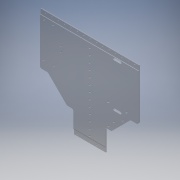
# Autodesk Inventor part: C15_TK_BatteryCrossStrut
Saved by Autodesk Inventor 2016 (Build 200138000, 138)
## iProperties
Created: 2016-01-20
Part Number: C15_TK_BatteryCrossStrut
Material: Polycarbonate, Clear
Document SubType Name: Modeling
Designer: TheeTimatahee
Density: 1.2 g/cm^3
Appearance: Polycarbonate - Clear
Mass: 810.244 g
Surface Area: 2322.62 cm^2
Volume: 675.204 cm^3
Author: TheeTimatahee
Autodesk Inventor part; units mm, degrees
ref_plane "YZ Plane" through (0, 0, 0) normal (1, 0, 0) x (0, 1, 0)
ref_plane "XZ Plane" through (0, 0, 0) normal (0, 1, 0) x (-1, 0, 0)
sketch "Sketch1" plane through (0, 0, 0) normal (0, 0, 1) x (1, 0, 0)
  line L0 (-196.85, -184.15) -> (196.85, -184.15)
  line L1 (196.85, -184.15) -> (196.85, 184.15)
  line L2 (196.85, 184.15) -> (-196.85, 184.15)
  line L3 (-196.85, 184.15) -> (-196.85, -184.15)
  line L4 (-196.85, -184.15) -> (196.85, 184.15) construction
  line L5 (196.85, -184.15) -> (-196.85, 184.15) construction
  point P0 (0, 0)
  dimension "d0" = 393.7
  dimension "d1" = 368.3
  constraints: 12 end point, 2 midpoint, 2 parallel, 1 horizontal, 1 perpendicular
  measures "d0" distance of L1.end L2.end
  measures "d1" distance of L0.end L1.end
extrude "Extrusion1" add sketch "Sketch1" along normal blind 6.35
sketch "Sketch2" plane through (0, 0, 6.35) normal (0, 0, 1) x (1, 0, 0)
  line L0 (-196.85, 184.15) -> (-196.85, -184.15) projected
  line L1 (-196.85, 165.1) -> (196.85, 165.1)
  line L2 (196.85, 165.1) -> (196.85, 184.15)
  line L3 (196.85, 184.15) -> (-196.85, 184.15)
  line L4 (-196.85, 184.15) -> (-196.85, 165.1)
  line L5 (-196.85, -184.15) -> (196.85, -184.15)
  line L6 (196.85, -184.15) -> (196.85, -165.1)
  line L7 (196.85, -165.1) -> (-196.85, -165.1)
  line L8 (-196.85, -165.1) -> (-196.85, -184.15)
  line L9 (196.85, -184.15) -> (196.85, 184.15) projected
  point P0 (0, 0)
  dimension "d4" = 330.2
  dimension "d5" = 19.05
  constraints: 16 end point, 4 parallel, 2 horizontal, 2 perpendicular, 1 collinear, 1 point on line
  measures "d4" distance between parallel lines of L7 L1
  measures "d5" distance between parallel lines of L3 L1
extrude "Extrusion2" cut sketch "Sketch2" against normal blind 2.54 contours L3 L2 L1 L0 | L7 L6 L5 L0
sketch "Sketch3" plane through (0, 0, 6.35) normal (0, 0, 1) x (1, 0, 0)
  line L0 (196.85, -184.15) -> (196.85, 165.1) projected
  line L1 (-196.85, 165.1) -> (-196.85, -165.1) projected
  line L2 (-63.5, -96.2801) -> (-63.5, -169.8131)
  line L3 (-196.85, -138.0631) -> (-196.85, -96.2801)
  line L4 (-169.0712, 11.938) -> (-156.3712, 11.938)
  line L5 (196.85, -184.15) -> (-196.85, -184.15) projected
  line L6 (-88.9, -96.2801) -> (-165.1, -20.0801)
  line L7 (-196.85, 184.15) -> (-196.85, -184.15) projected
  line L8 (-63.5, -96.2801) -> (-196.85, -96.2801)
  line L9 (-196.85, -96.2801) -> (-196.85, -7.3801)
  line L10 (-63.5, -169.8131) -> (-63.5, -184.15)
  line L11 (-63.5, -169.8131) -> (-63.5, -169.8131)
  line L12 (176.1744, -166.6059) -> (83.0336, -166.6059)
  line L13 (-176.1744, -166.6381) -> (-83.0336, -166.6381)
  line L14 (-176.1744, -102.6301) -> (-83.0336, -102.6301)
  line L15 (176.1744, -102.5979) -> (83.0336, -102.5979)
  line L16 (0, -214.5967) -> (0, 32.3311)
  line L17 (196.85, 165.1) -> (196.85, -165.1)
  line L18 (63.5, -96.2801) -> (63.5, -169.8131)
  line L19 (88.9, -96.2801) -> (165.1, -20.0801)
  line L20 (63.5, -96.2801) -> (196.85, -96.2801)
  line L21 (63.5, -169.8131) -> (63.5, -184.15)
  line L22 (63.5, -169.8131) -> (63.5, -169.8131)
  line L23 (196.85, -165.1) -> (196.85, -184.15)
  line L24 (196.85, -184.15) -> (196.85, 184.15) projected
  line L25 (196.85, -184.15) -> (63.5, -184.15)
  line L26 (-63.5, -184.15) -> (-196.85, -184.15)
  line L27 (-196.85, -184.15) -> (196.85, -184.15) projected
  line L28 (-196.85, -184.15) -> (-196.85, -138.0631)
  line L29 (-196.85, -20.0801) -> (196.85, -20.0801)
  line L30 (-196.85, -96.2801) -> (-196.85, -20.0801)
  line L31 (-196.85, -20.0801) -> (-165.1, -20.0801)
  line L32 (-165.1, -20.0801) -> (-165.1, -96.2801)
  line L33 (-165.1, -96.2801) -> (-196.85, -96.2801)
  line L34 (-196.85, -96.2801) -> (-196.85, -20.0801)
  point P0 (0, 0)
  point P1 (101.6, -190.5)
  dimension "d45" = 45
  dimension "d47" = 6.35
  dimension "d48" = 3.175
  dimension "d49" = 25.4
  dimension "d50" = 45
  dimension "d51" = 76.2
  constraints: 58 end point, 10 point on line, 9 horizontal, 7 symmetric about line, 5 collinear, 3 parallel, 3 perpendicular, 3 vertical, 13 other
  measures "d45" angle of L6 L8
  measures "d47" distance between parallel lines of L14 L8
  measures "d48" distance between parallel lines of L11 L13
  measures "d49" distance from line of L2 L6.start
  measures "d50" angle of L20 L19
  measures "d51" distance between parallel lines of L20 L29
extrude "Extrusion3" cut sketch "Sketch3" against normal through all contours L5 L21 L18 L20 L0 | L20 L19 L29 L0 | L5 L7 L1 L8 L2 L10 | L32 L8 L1 L29 | L6 L8 L32
fillet "Fillet1" radius 6.35 8 edges at (-88.9, -96.2801, 3.175) (-63.5, -96.2801, 3.175) (-165.1, -20.0801, 3.175) (-196.85, -20.0801, 3.175) (63.5, -96.2801, 3.175) (88.9, -96.2801, 3.175) (165.1, -20.0801, 3.175) (196.85, -20.0801, 3.175)
sketch "Sketch5" plane through (0, 0, 0) normal (0, 0, -1) x (-1, 0, 0)
  line L0 (63.5, -184.15) -> (63.5, -102.6301) projected
  line L1 (-196.85, 184.15) -> (196.85, 184.15) projected
  line L2 (196.85, 184.15) -> (196.85, -13.7301) projected
  point P0 (0, 0)
  point P1 (50.8, -177.8)
  point P2 (63.5, -163.4631)
  point P3 (177.8, 177.8)
  point P4 (152.4, 177.8)
  point P5 (127, 177.8)
  point P6 (101.6, 177.8)
  point P7 (76.2, 177.8)
  point P8 (50.8, 177.8)
  point P9 (25.4, 177.8)
  point P10 (0, 177.8)
  point P11 (-25.4, 177.8)
  point P12 (-50.8, 177.8)
  point P13 (-76.2, 177.8)
  point P14 (-101.6, 177.8)
  point P15 (-127, 177.8)
  point P16 (-152.4, 177.8)
  point P17 (-177.8, 177.8)
  point P18 (25.4, -177.8)
  point P19 (0, -177.8)
  point P20 (-25.4, -177.8)
  point P21 (-50.8, -177.8)
  dimension "d100" = 12.7
  dimension "d101" = 6.35
  dimension "d102" = 19.05
  dimension "d105" = 25.4
  dimension "d112" = 25.4
  constraints: 2 horizontal, 18 other
  measures "d100" distance from line of L0 point (50.8, -177.8)
  measures "d101" distance from line of L1 point (177.8, 177.8)
  measures "d102" distance from line of L2 point (177.8, 177.8)
  measures "d105" distance of point (177.8, 177.8) point (152.4, 177.8)
  measures "d112" distance of point (50.8, -177.8) point (25.4, -177.8)
hole "Hole2" at (-177.8, 177.8, 0) at (-152.4, 177.8, 0) at (-127, 177.8, 0) at (-101.6, 177.8, 0) at (-76.2, 177.8, 0) at (-50.8, 177.8, 0) at (-25.4, 177.8, 0) at (0, 177.8, 0) at (25.4, 177.8, 0) at (50.8, 177.8, 0) at (76.2, 177.8, 0) at (101.6, 177.8, 0) at (127, 177.8, 0) at (152.4, 177.8, 0) at (177.8, 177.8, 0) at (-50.8, -177.8, 0) at (-25.4, -177.8, 0) at (0, -177.8, 0) at (25.4, -177.8, 0) at (50.8, -177.8, 0) direction (0, 0, 1) diameter 4.1402 end through all
sketch "Sketch6" plane through (0, 0, 0) normal (0, 0, -1) x (-1, 0, 0)
  circle A0 centre (145.669, 153.0766) radius 2.4116 projected
  circle A1 centre (181.737, 153.0766) radius 2.4116 projected
  circle A2 centre (143.256, 13.1318) radius 2.4116 projected
  circle A3 centre (184.15, 13.1318) radius 2.4116 projected
  point P0 (0, 0)
hole "Hole3" at (-143.256, 13.1318, 0) at (-184.15, 13.1318, 0) at (-145.669, 153.0766, 0) at (-181.737, 153.0766, 0) direction (0, 0, 1) diameter 4.826 end through all
sketch "Sketch7" plane through (0, 0, 0) normal (0, 0, -1) x (-1, 0, 0)
  circle A0 centre (0, 184.15) radius 2.0701 projected
  line L0 (-9.6012, -190.5) -> (9.6012, -190.5) projected
  line L1 (9.6012, 190.5) -> (9.6012, -190.5) projected
  line L2 (9.6012, 190.5) -> (-9.6012, 190.5) projected
  line L3 (-9.6012, -190.5) -> (-9.6012, 190.5) projected
  circle A1 centre (0, 171.45) radius 2.0701 projected
  circle A2 centre (0, 146.05) radius 2.0701 projected
  circle A3 centre (0, 120.65) radius 2.0701 projected
  circle A4 centre (0, 95.25) radius 2.0701 projected
  circle A5 centre (0, 69.85) radius 2.0701 projected
  circle A6 centre (0, 44.45) radius 2.0701 projected
  circle A7 centre (0, 19.05) radius 2.0701 projected
  circle A8 centre (0, -6.35) radius 2.0701 projected
  circle A9 centre (0, -31.75) radius 2.0701 projected
  circle A10 centre (0, -57.15) radius 2.0701 projected
  circle A11 centre (0, -82.55) radius 2.0701 projected
  circle A12 centre (0, -107.95) radius 2.0701 projected
  circle A13 centre (0, -133.35) radius 2.0701 projected
  circle A14 centre (0, -158.75) radius 2.0701 projected
  circle A15 centre (0, -184.15) radius 2.0701 projected
  line L4 (-196.85, 165.1) -> (196.85, 165.1) projected
  line L5 (-36.3783, -2.794) -> (-171.9439, -2.794)
  line L6 (-123.19, -16.002) -> (-97.79, -16.002) construction
  line L7 (-123.19, -20.828) -> (-97.79, -20.828)
  line L8 (-97.79, -11.176) -> (-123.19, -11.176)
  arc A16 (-123.19, -11.176) -> (-123.19, -20.828) centre (-123.19, -16.002) ccw
  arc A17 (-97.79, -20.828) -> (-97.79, -11.176) centre (-97.79, -16.002) ccw
  line L9 (-123.19, 158.75) -> (-97.79, 158.75) construction
  line L10 (-123.19, 153.924) -> (-97.79, 153.924)
  line L11 (-97.79, 163.576) -> (-123.19, 163.576)
  arc A18 (-123.19, 163.576) -> (-123.19, 153.924) centre (-123.19, 158.75) ccw
  arc A19 (-97.79, 153.924) -> (-97.79, 163.576) centre (-97.79, 158.75) ccw
  line L12 (-110.49, 207.2769) -> (-110.49, -6.4547)
  line L13 (-196.85, -13.7301) -> (-196.85, 165.1) projected
  point P0 (0, 0)
  point P1 (-74.295, -2.794)
  point P2 (-146.685, -2.794)
  point P3 (-110.49, -16.002)
  point P4 (-110.49, 158.75)
  dimension "d118" = 72.39
  dimension "d119" = 13.208
  dimension "d120" = 4.826
  dimension "d121" = 25.4
  dimension "d122" = 23.495
  dimension "d123" = 4.826
  dimension "d124" = 25.4
  dimension "d127" = 6.35
  dimension "d128" = 86.36
  dimension "d129" = 165.1
  constraints: 20 end point, 8 point on circle, 8 tangent, 4 centre point, 4 point on line, 3 horizontal, 2 midpoint, 2 parallel, 1 vertical
  measures "d118" distance of point (-146.685, -2.794) point (-74.295, -2.794)
  measures "d119" distance from line of L5 point (-110.49, -16.002)
  measures "d120" radius of A17
  measures "d121" distance of L6.end L6.start
  measures "d122" horizontal distance of point (-74.295, -2.794) L6.end
  measures "d123" radius of A19
  measures "d124" distance of L9.start L9.end
  measures "d127" distance from line of L4 point (-110.49, 158.75)
  measures "d128" distance between parallel lines of L13 L12
  measures "d129" distance between parallel lines of L8 L10
extrude "Extrusion4" cut sketch "Sketch7" against normal through all contours L11 A19 L10 L12 | L12 L10 A18 L11 | A16 L8 A17 L7
hole "Hole4" at (74.295, -2.794, 0) at (146.685, -2.794, 0) direction (0, 0, 1) diameter 6.858 end through all
hole "Hole6" at (0, 146.05, 0) at (0, 120.65, 0) at (0, 95.25, 0) at (0, 69.85, 0) at (0, 44.45, 0) at (0, 19.05, 0) at (0, -6.35, 0) at (0, -31.75, 0) at (0, -57.15, 0) at (0, -82.55, 0) at (0, -107.95, 0) at (0, -133.35, 0) at (0, -158.75, 0) direction (0, 0, 1) diameter 5.1054 end through all clearance for "Flat Head Machine Screw (82)" size "#10" standard "Ansi Unified Screw Threads"
ref_plane "Work Plane1" through (0, 0, 3.175) normal (0, 0, -1) x (-1, 0, 0)
sketch "Sketch8" plane through (0, 0, 3.175) normal (0, 0, -1) x (-1, 0, 0)
  circle A0 centre (0, -133.35) radius 2.5527 projected
  circle A1 centre (0, -82.55) radius 2.5527 projected
  circle A2 centre (0, -31.75) radius 2.5527 projected
  circle A3 centre (0, 19.05) radius 2.5527 projected
  circle A4 centre (0, 69.85) radius 2.5527 projected
  circle A5 centre (0, 120.65) radius 2.5527 projected
  circle A6 centre (0, 146.05) radius 2.5527 projected
  circle A7 centre (0, 95.25) radius 2.5527 projected
  circle A8 centre (0, 44.45) radius 2.5527 projected
  circle A9 centre (0, -6.35) radius 2.5527 projected
  circle A10 centre (0, -57.15) radius 2.5527 projected
  circle A11 centre (0, -107.95) radius 2.5527 projected
  circle A12 centre (0, -158.75) radius 2.5527 projected
  circle A13 centre (145.669, 153.0766) radius 2.413 projected
  circle A14 centre (143.256, 13.1318) radius 2.413 projected
  circle A15 centre (184.15, 13.1318) radius 2.413 projected
  circle A16 centre (181.737, 153.0766) radius 2.413 projected
  circle A17 centre (-25.4, -177.8) radius 2.0701 projected
  circle A18 centre (25.4, -177.8) radius 2.0701 projected
  circle A19 centre (-177.8, 177.8) radius 2.0701 projected
  circle A20 centre (-127, 177.8) radius 2.0701 projected
  circle A21 centre (-76.2, 177.8) radius 2.0701 projected
  circle A22 centre (-25.4, 177.8) radius 2.0701 projected
  circle A23 centre (25.4, 177.8) radius 2.0701 projected
  circle A24 centre (76.2, 177.8) radius 2.0701 projected
  circle A25 centre (127, 177.8) radius 2.0701 projected
  circle A26 centre (177.8, 177.8) radius 2.0701 projected
  circle A27 centre (152.4, 177.8) radius 2.0701 projected
  circle A28 centre (101.6, 177.8) radius 2.0701 projected
  circle A29 centre (50.8, 177.8) radius 2.0701 projected
  circle A30 centre (0, 177.8) radius 2.0701 projected
  circle A31 centre (-50.8, 177.8) radius 2.0701 projected
  circle A32 centre (-101.6, 177.8) radius 2.0701 projected
  circle A33 centre (-152.4, 177.8) radius 2.0701 projected
  circle A34 centre (50.8, -177.8) radius 2.0701 projected
  circle A35 centre (0, -177.8) radius 2.0701 projected
  circle A36 centre (-50.8, -177.8) radius 2.0701 projected
  arc A37 (-196.85, -13.7301) -> (-190.5, -20.0801) centre (-190.5, -13.7301) ccw projected
  line L0 (-190.5, -20.0801) -> (-167.7303, -20.0801) projected
  arc A38 (-163.2401, -21.9399) -> (-167.7303, -20.0801) centre (-167.7303, -26.4301) ccw projected
  line L1 (-163.2401, -21.9399) -> (-90.7599, -94.4202) projected
  arc A39 (-90.7599, -94.4202) -> (-86.2697, -96.2801) centre (-86.2697, -89.9301) ccw projected
  line L2 (-86.2697, -96.2801) -> (-69.85, -96.2801) projected
  arc A40 (-63.5, -102.6301) -> (-69.85, -96.2801) centre (-69.85, -102.6301) ccw projected
  line L3 (-63.5, -102.6301) -> (-63.5, -184.15) projected
  line L4 (63.5, -184.15) -> (-63.5, -184.15) projected
  line L5 (63.5, -184.15) -> (63.5, -102.6301) projected
  arc A41 (69.85, -96.2801) -> (63.5, -102.6301) centre (69.85, -102.6301) ccw projected
  line L6 (69.85, -96.2801) -> (86.2697, -96.2801) projected
  arc A42 (86.2697, -96.2801) -> (90.7599, -94.4202) centre (86.2697, -89.9301) ccw projected
  line L7 (90.7599, -94.4202) -> (163.2401, -21.9399) projected
  arc A43 (167.7303, -20.0801) -> (163.2401, -21.9399) centre (167.7303, -26.4301) ccw projected
  line L8 (167.7303, -20.0801) -> (190.5, -20.0801) projected
  arc A44 (190.5, -20.0801) -> (196.85, -13.7301) centre (190.5, -13.7301) ccw projected
  line L9 (196.85, 184.15) -> (196.85, -13.7301) projected
  line L10 (-196.85, 184.15) -> (196.85, 184.15) projected
  line L11 (-196.85, -13.7301) -> (-196.85, 184.15) projected
  circle A45 centre (0, -133.35) radius 2.5527 projected
  circle A46 centre (0, -82.55) radius 2.5527 projected
  circle A47 centre (0, -31.75) radius 2.5527 projected
  circle A48 centre (0, 19.05) radius 2.5527 projected
  circle A49 centre (0, 69.85) radius 2.5527 projected
  circle A50 centre (0, 120.65) radius 2.5527 projected
  circle A51 centre (0, 146.05) radius 2.5527 projected
  circle A52 centre (0, 95.25) radius 2.5527 projected
  circle A53 centre (0, 44.45) radius 2.5527 projected
  circle A54 centre (0, -6.35) radius 2.5527 projected
  circle A55 centre (0, -57.15) radius 2.5527 projected
  circle A56 centre (0, -107.95) radius 2.5527 projected
  circle A57 centre (0, -158.75) radius 2.5527 projected
  circle A58 centre (145.669, 153.0766) radius 2.413 projected
  circle A59 centre (143.256, 13.1318) radius 2.413 projected
  circle A60 centre (184.15, 13.1318) radius 2.413 projected
  circle A61 centre (181.737, 153.0766) radius 2.413 projected
  arc A62 (-196.85, -13.7301) -> (-190.5, -20.0801) centre (-190.5, -13.7301) ccw projected
  line L12 (-196.85, -13.7301) -> (-196.85, 165.1) projected
  line L13 (-196.85, 165.1) -> (196.85, 165.1) projected
  line L14 (196.85, 165.1) -> (196.85, -13.7301) projected
  arc A63 (190.5, -20.0801) -> (196.85, -13.7301) centre (190.5, -13.7301) ccw projected
  line L15 (190.5, -20.0801) -> (167.7303, -20.0801) projected
  arc A64 (167.7303, -20.0801) -> (163.2401, -21.9399) centre (167.7303, -26.4301) ccw projected
  line L16 (163.2401, -21.9399) -> (90.7599, -94.4202) projected
  arc A65 (86.2697, -96.2801) -> (90.7599, -94.4202) centre (86.2697, -89.9301) ccw projected
  line L17 (86.2697, -96.2801) -> (69.85, -96.2801) projected
  arc A66 (69.85, -96.2801) -> (63.5, -102.6301) centre (69.85, -102.6301) ccw projected
  line L18 (63.5, -102.6301) -> (63.5, -165.1) projected
  line L19 (63.5, -165.1) -> (-63.5, -165.1) projected
  line L20 (-63.5, -165.1) -> (-63.5, -102.6301) projected
  arc A67 (-63.5, -102.6301) -> (-69.85, -96.2801) centre (-69.85, -102.6301) ccw projected
  line L21 (-69.85, -96.2801) -> (-86.2697, -96.2801) projected
  arc A68 (-90.7599, -94.4202) -> (-86.2697, -96.2801) centre (-86.2697, -89.9301) ccw projected
  line L22 (-90.7599, -94.4202) -> (-163.2401, -21.9399) projected
  arc A69 (-163.2401, -21.9399) -> (-167.7303, -20.0801) centre (-167.7303, -26.4301) ccw projected
  line L23 (-167.7303, -20.0801) -> (-190.5, -20.0801) projected
  line L24 (89.15, 101.9) -> (89.15, 107.9) projected
  line L25 (89.15, 101.9) -> (85.65, 101.9) projected
  line L26 (85.65, 60.9) -> (85.65, 101.9) projected
  line L27 (120.65, 60.9) -> (85.65, 60.9) projected
  line L28 (120.65, 110.9) -> (120.65, 60.9) projected
  line L29 (85.65, 110.9) -> (120.65, 110.9) projected
  line L30 (85.65, 107.9) -> (85.65, 110.9) projected
  line L31 (89.15, 107.9) -> (85.65, 107.9) projected
  circle A70 centre (113.65, 95.9) radius 2.15 projected
  circle A71 centre (113.65, 75.9) radius 2.15 projected
  point P0 (0, 0)
sketch "Sketch9" plane through (0, 0, 6.35) normal (0, 0, 1) x (1, 0, 0)
  arc A0 (168.4147, -77.5476) -> (161.6583, -77.5476) centre (165.0365, -77.5476) ccw projected
  line L0 (168.4147, -77.5476) -> (168.4147, -80.7226) projected
  arc A1 (161.6583, -80.7226) -> (168.4147, -80.7226) centre (165.0365, -80.7226) ccw projected
  line L1 (161.6583, -80.7226) -> (161.6583, -77.5476) projected
  line L2 (182.8165, -99.4551) -> (55.8165, -99.4551) projected
  line L3 (182.8165, -29.6051) -> (182.8165, -99.4551) projected
  line L4 (128.7395, -29.6051) -> (182.8165, -29.6051) projected
  line L5 (55.8165, -80.6663) -> (128.7395, -29.6051) projected
  line L6 (55.8165, -99.4551) -> (55.8165, -80.6663) projected
  circle A2 centre (97.0915, -61.3551) radius 2.5527 projected
  circle A3 centre (74.8665, -86.7551) radius 2.5527 projected
  circle A4 centre (132.0292, -39.1301) radius 2.5527 projected
hole "Hole7" at (132.0292, -39.1301, 6.35) at (97.0915, -61.3551, 6.35) at (74.8665, -86.7551, 6.35) direction (0, 0, -1) diameter 5.1054 end through all clearance for "Flat Head Machine Screw (82)" size "#10" standard "Ansi Unified Screw Threads"
hole "Hole8" at (-113.65, 75.9, 3.175) at (-113.65, 95.9, 3.175) direction (0, 0, 1) diameter 4.2926 end through all
sketch "Sketch10" plane through (0, 0, 6.35) normal (0, 0, 1) x (1, 0, 0)
  circle A0 centre (-113.65, 75.9) radius 2.1463 projected
  circle A1 centre (-113.65, 95.9) radius 2.1463 projected
  circle A2 centre (97.0915, -61.3551) radius 2.5527 projected
  circle A3 centre (132.0292, -39.1301) radius 2.5527 projected
  circle A4 centre (74.8665, -86.7551) radius 2.5527 projected
  circle A5 centre (0, -133.35) radius 2.5527 projected
  circle A6 centre (0, -82.55) radius 2.5527 projected
  circle A7 centre (0, -31.75) radius 2.5527 projected
  circle A8 centre (0, 19.05) radius 2.5527 projected
  circle A9 centre (0, 69.85) radius 2.5527 projected
  circle A10 centre (0, 120.65) radius 2.5527 projected
  circle A11 centre (0, 146.05) radius 2.5527 projected
  circle A12 centre (0, 95.25) radius 2.5527 projected
  circle A13 centre (0, 44.45) radius 2.5527 projected
  circle A14 centre (0, -6.35) radius 2.5527 projected
  circle A15 centre (0, -57.15) radius 2.5527 projected
  circle A16 centre (0, -107.95) radius 2.5527 projected
  circle A17 centre (0, -158.75) radius 2.5527 projected
  circle A18 centre (74.295, -2.794) radius 3.429 projected
  circle A19 centre (146.685, -2.794) radius 3.429 projected
  arc A20 (97.79, -11.176) -> (97.79, -20.828) centre (97.79, -16.002) ccw projected
  line L0 (97.79, -11.176) -> (123.19, -11.176) projected
  arc A21 (123.19, -20.828) -> (123.19, -11.176) centre (123.19, -16.002) ccw projected
  line L1 (123.19, -20.828) -> (97.79, -20.828) projected
  arc A22 (97.79, 163.576) -> (97.79, 153.924) centre (97.79, 158.75) ccw projected
  line L2 (97.79, 163.576) -> (123.19, 163.576) projected
  arc A23 (123.19, 153.924) -> (123.19, 163.576) centre (123.19, 158.75) ccw projected
  line L3 (123.19, 153.924) -> (97.79, 153.924) projected
  circle A24 centre (-145.669, 153.0766) radius 2.413 projected
  circle A25 centre (-143.256, 13.1318) radius 2.413 projected
  circle A26 centre (-184.15, 13.1318) radius 2.413 projected
  circle A27 centre (-181.737, 153.0766) radius 2.413 projected
  arc A28 (190.5, -20.0801) -> (196.85, -13.7301) centre (190.5, -13.7301) ccw projected
  line L4 (196.85, -13.7301) -> (196.85, 165.1) projected
  line L5 (196.85, 165.1) -> (-196.85, 165.1) projected
  line L6 (-196.85, 165.1) -> (-196.85, -13.7301) projected
  arc A29 (-196.85, -13.7301) -> (-190.5, -20.0801) centre (-190.5, -13.7301) ccw projected
  line L7 (-190.5, -20.0801) -> (-167.7303, -20.0801) projected
  arc A30 (-163.2401, -21.9399) -> (-167.7303, -20.0801) centre (-167.7303, -26.4301) ccw projected
  line L8 (-163.2401, -21.9399) -> (-90.7599, -94.4202) projected
  arc A31 (-90.7599, -94.4202) -> (-86.2697, -96.2801) centre (-86.2697, -89.9301) ccw projected
  line L9 (-86.2697, -96.2801) -> (-69.85, -96.2801) projected
  arc A32 (-63.5, -102.6301) -> (-69.85, -96.2801) centre (-69.85, -102.6301) ccw projected
  line L10 (-63.5, -102.6301) -> (-63.5, -165.1) projected
  line L11 (-63.5, -165.1) -> (63.5, -165.1) projected
  line L12 (63.5, -165.1) -> (63.5, -102.6301) projected
  arc A33 (69.85, -96.2801) -> (63.5, -102.6301) centre (69.85, -102.6301) ccw projected
  line L13 (69.85, -96.2801) -> (86.2697, -96.2801) projected
  arc A34 (86.2697, -96.2801) -> (90.7599, -94.4202) centre (86.2697, -89.9301) ccw projected
  line L14 (90.7599, -94.4202) -> (163.2401, -21.9399) projected
  arc A35 (167.7303, -20.0801) -> (163.2401, -21.9399) centre (167.7303, -26.4301) ccw projected
  line L15 (167.7303, -20.0801) -> (190.5, -20.0801) projected
  circle A36 centre (177.8, 177.8) radius 2.0701 projected
  circle A37 centre (127, 177.8) radius 2.0701 projected
  circle A38 centre (76.2, 177.8) radius 2.0701 projected
  circle A39 centre (25.4, 177.8) radius 2.0701 projected
  circle A40 centre (-25.4, 177.8) radius 2.0701 projected
  circle A41 centre (-76.2, 177.8) radius 2.0701 projected
  circle A42 centre (-127, 177.8) radius 2.0701 projected
  circle A43 centre (-177.8, 177.8) radius 2.0701 projected
  circle A44 centre (-152.4, 177.8) radius 2.0701 projected
  circle A45 centre (-101.6, 177.8) radius 2.0701 projected
  circle A46 centre (-50.8, 177.8) radius 2.0701 projected
  circle A47 centre (0, 177.8) radius 2.0701 projected
  circle A48 centre (50.8, 177.8) radius 2.0701 projected
  circle A49 centre (101.6, 177.8) radius 2.0701 projected
  circle A50 centre (152.4, 177.8) radius 2.0701 projected
  line L16 (196.85, 165.1) -> (-196.85, 165.1) projected
  line L17 (196.85, 184.15) -> (196.85, 165.1) projected
  line L18 (-196.85, 184.15) -> (196.85, 184.15) projected
  line L19 (-196.85, 165.1) -> (-196.85, 184.15) projected
  circle A51 centre (25.4, -177.8) radius 2.0701 projected
  circle A52 centre (-25.4, -177.8) radius 2.0701 projected
  circle A53 centre (-50.8, -177.8) radius 2.0701 projected
  circle A54 centre (0, -177.8) radius 2.0701 projected
  circle A55 centre (50.8, -177.8) radius 2.0701 projected
  line L20 (-63.5, -165.1) -> (-63.5, -184.15) projected
  line L21 (63.5, -184.15) -> (-63.5, -184.15) projected
  line L22 (63.5, -184.15) -> (63.5, -165.1) projected
  line L23 (-63.5, -165.1) -> (63.5, -165.1) projected
  point P0 (0, 0)
body "Solid1"
